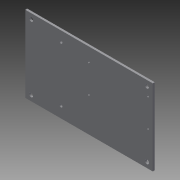
# Autodesk Inventor part: base_ps
Saved by Autodesk Inventor 2014 (Build 180170000, 170)
## iProperties
Created: 2015-04-20
Part Number: base_ps
Material: Generic
Document SubType Name: Modeling
Designer: Sousaadm
Density: 1 g/cm^3
Appearance: Default
Author: Sousaadm
Autodesk Inventor part; units mm, degrees
ref_plane "YZ Plane" through (0, 0, 0) normal (1, 0, 0) x (0, 1, 0)
ref_plane "XZ Plane" through (0, 0, 0) normal (0, 1, 0) x (-1, 0, 0)
ref_plane "XY Plane" through (0, 0, 0) normal (0, 0, 1) x (1, 0, 0)
sketch "Sketch1" plane through (0, 0, 0) normal (0, 1, 0) x (-1, 0, 0)
  line L0 (0, 0) -> (-127, 0)
  line L1 (-127, 0) -> (-127, 76)
  line L2 (-127, 76) -> (0, 76)
  line L3 (0, 76) -> (0, 0)
  dimension "d0" = 76
  dimension "d1" = 127
  constraints: 8 end point, 2 parallel, 1 horizontal, 1 perpendicular
  measures "d0" distance of L2.end L0.start
  measures "d1" distance of L1.end L2.end
extrude "Extrusion1" add sketch "Sketch1" along normal blind 2
sketch "Sketch2" plane through (0, 0, 0) normal (0, -1, 0) x (1, 0, 0)
  line L0 (0, 0) -> (127, 0) projected
  line L1 (127, 0) -> (127, 76) projected
  line L2 (127, 76) -> (0, 76) projected
  line L3 (0, 76) -> (0, 0) projected
  line L4 (0, 5.4) -> (127, 5.4) construction
  line L5 (0, 38) -> (127, 38) construction
  line L6 (63.5, 76) -> (63.5, 0) construction
  line L7 (121.2, 76) -> (121.2, 0) construction
  line L8 (0, 70.6) -> (127, 70.6) construction
  line L9 (5.8, 76) -> (5.8, 0) construction
  circle A0 centre (121.2, 70.6) radius 2
  circle A1 centre (121.2, 5.4) radius 2
  circle A2 centre (5.8, 70.6) radius 2
  circle A3 centre (5.8, 5.4) radius 2
  dimension "d5" = 32.6
  dimension "d6" = 57.7
  dimension "d7" = 4
  constraints: 12 end point, 7 symmetric about line, 6 point on line, 4 centre point, 4 midpoint, 2 perpendicular, 3 other
  measures "d5" distance between parallel lines of L4 L5
  measures "d6" distance between parallel lines of L7 L6
  measures "d7" diameter of A0
extrude "Extrusion2" cut sketch "Sketch2" against normal through all contours A0 | A1 | A2 | A3
sketch "Sketch3" plane through (0, 0, 0) normal (0, -1, 0) x (1, 0, 0)
  line L0 (0, 0) -> (127, 0) projected
  line L1 (0, 76) -> (0, 0) projected
  line L2 (10, 93) -> (61, 93)
  line L3 (61, 93) -> (61, 0)
  line L4 (61, 0) -> (10, 0)
  line L5 (10, 0) -> (10, 93)
  line L6 (61, 32) -> (124, 32)
  line L7 (124, 32) -> (124, 67)
  line L8 (124, 67) -> (61, 67)
  line L9 (61, 67) -> (61, 32)
  line L10 (35.5, 93) -> (35.5, 0) construction
  circle A0 centre (35.5, 11) radius 1.5
  circle A1 centre (35.5, 66) radius 1.5
  line L11 (92.5, 67) -> (92.5, 32) construction
  line L12 (124, 49.5) -> (61, 49.5) construction
  circle A2 centre (122, 34.5) radius 1
  circle A3 centre (122, 62.5) radius 1
  circle A4 centre (63.1, 34.5) radius 1
  circle A5 centre (63.1, 62.5) radius 1
  dimension "d10" = 93
  dimension "d12" = 51
  dimension "d13" = 10
  dimension "d14" = 63
  dimension "d15" = 35
  dimension "d16" = 11
  dimension "d17" = 3
  dimension "d20" = 55
  dimension "d25" = 32
  dimension "d26" = 29.5
  dimension "d27" = 2
  dimension "d28" = 15
  dimension "d31" = 28
  dimension "d34" = 58.9
  constraints: 22 end point, 6 centre point, 6 midpoint, 4 parallel, 3 horizontal, 2 collinear, 2 perpendicular, 2 vertical, 1 point on line, 8 other
  measures "d10" distance of L4.end L2.start
  measures "d12" distance of L2.start L2.end
  measures "d13" distance between parallel lines of L1 L5
  measures "d14" distance of L7.end L8.end
  measures "d15" distance of L6.end L7.end
  measures "d16" distance from line of L0 A0.centre
  measures "d17" diameter of A0
  measures "d20" distance of A0.centre A1.centre
  measures "d25" distance between parallel lines of L0 L6
  measures "d26" distance from line of A2.centre L11
  measures "d27" diameter of A2
  measures "d28" distance from line of A2.centre L12
  measures "d31" distance of A2.centre A3.centre
  measures "d34" distance of A2.centre A4.centre
extrude "Extrusion3" cut sketch "Sketch3" against normal through all contours A0 | A1 | A2 | A3 | A4 | A5
body "Solid1"
